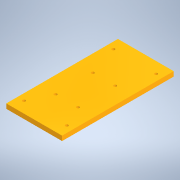
# Autodesk Inventor part: bottom_plate
Saved by Autodesk Inventor 2020 (Build 240168000, 168)
## iProperties
Created: 2021-04-04
Part Number: bottom_plate
Material: PET Plastic
Document SubType Name: Modeling
Designer: Devin
Density: 1.541 g/cm^3
Appearance: Smooth - Light Orange
Author: Devin
Autodesk Inventor part; units mm, degrees
ref_plane "YZ Plane" through (0, 0, 0) normal (1, 0, 0) x (0, 1, 0)
ref_plane "XZ Plane" through (0, 0, 0) normal (0, 1, 0) x (-1, 0, 0)
ref_plane "XY Plane" through (0, 0, 0) normal (0, 0, 1) x (1, 0, 0)
sketch "Sketch1" plane through (0, 0, 0) normal (0, 1, 0) x (-1, 0, 0)
  line L0 (0, 0) -> (60, 0)
  line L1 (60, 0) -> (60, -120)
  line L2 (60, -120) -> (0, -120)
  line L3 (0, -120) -> (0, 0)
  dimension "d0" = 60
  dimension "d1" = 120
  constraints: 8 end point, 2 parallel, 1 horizontal, 1 perpendicular
  measures "d0" distance of L0.start L0.end
  measures "d1" distance of L0.end L1.end
extrude "Extrusion1" add sketch "Sketch1" along normal blind 5
sketch "Sketch3" plane through (-60, 0, 0) normal (0, 0, 1) x (1, 0, 0)
  line L0 (0, 0) -> (60, 0) projected
  circle A0 centre (38.75, 11) radius 1.55
  circle A1 centre (21.25, 11) radius 1.55
  dimension "d22" = 3.1
  dimension "d23" = 3.1
  dimension "d25" = 17.5
  dimension "d26" = 11
  dimension "d27" = 11
  constraints: 2 centre point
  measures "d22" diameter of A0
  measures "d23" diameter of A1
  measures "d25" distance of A0.centre A1.centre
  measures "d26" distance from line of L0 A1.centre
  measures "d27" distance from line of L0 A0.centre
extrude "Extrusion3" cut sketch "Sketch3" against normal through all
sketch "Sketch5" plane through (0, 5, 0) normal (0, 1, 0) x (1, 0, 0)
  line L0 (0, 0) -> (0, 120) projected
  line L1 (0, 120) -> (0, 108)
  line L2 (0, 108) -> (-7, 108)
  line L3 (-60, 120) -> (-60, 0) projected
  circle A0 centre (-7, 108) radius 1.55
  line L4 (0, 120) -> (-60, 120) projected
  line L5 (-30, 120) -> (-30, 0)
  line L6 (-45, 0) -> (-15, 0) projected
  line L7 (0, 60) -> (-60, 60)
  circle A1 centre (-53, 108) radius 1.55
  circle A2 centre (-7, 12) radius 1.55
  circle A3 centre (-53, 12) radius 1.55
  dimension "d47" = 12
  dimension "d48" = 7
  dimension "d49" = 3.1
  constraints: 8 end point, 4 centre point, 4 midpoint, 3 symmetric about line, 1 coincident, 1 perpendicular, 1 point on line, 3 other
  measures "d47" distance of L0.end L1.end
  measures "d48" distance of L1.end L2.end
  measures "d49" diameter of A0
extrude "Extrusion5" cut sketch "Sketch5" against normal blind 10 contours A0 | A1 | A2 | A3
sketch "Sketch7" plane through (0, 5, 0) normal (0, 1, 0) x (1, 0, 0)
  circle A0 centre (-18, 75) radius 2.45 projected
  circle A1 centre (-42, 75) radius 2.45 projected
  circle A2 centre (-42, 35) radius 2.45 projected
  circle A3 centre (-18, 35) radius 2.45 projected
  circle A4 centre (-18, 35) radius 1.55
  circle A5 centre (-42, 35) radius 1.55
  circle A6 centre (-18, 75) radius 1.55
  circle A7 centre (-42, 75) radius 1.55
  point P0 (0, 0)
  dimension "d64" = 3.1
  dimension "d65" = 3.1
  dimension "d66" = 3.1
  dimension "d67" = 3.1
  constraints: 4 centre point, 4 coincident
  measures "d64" diameter of A4
  measures "d65" diameter of A5
  measures "d66" diameter of A6
  measures "d67" diameter of A7
extrude "Extrusion7" cut sketch "Sketch7" against normal blind 10 contours A4 | A5 | A6 | A7
body "Solid1"
